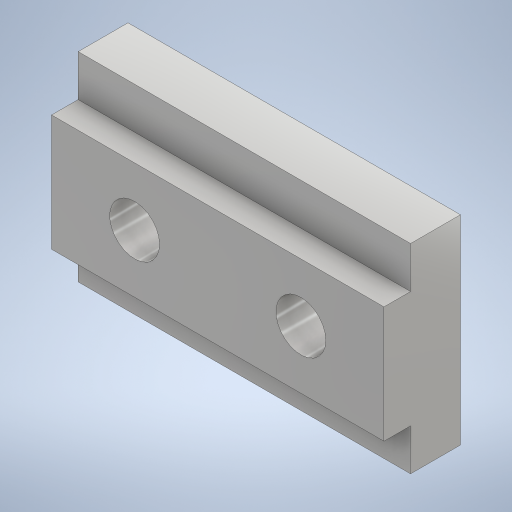
# Autodesk Inventor part: slider2b
Saved by Autodesk Inventor 2024.1 (Build 281209000, 209)
## iProperties
Created: 2017-08-05
Part Number: slider2b
Material: アルミニウム 6061-AHC
Document SubType Name: Modeling
Designer: SHUICHI
Density: 2.7 g/cm^3
Appearance: アルミニウム - ダーク
Mass: 2.37322 g
Surface Area: 8.16834 cm^2
Volume: 0.878969 cm^3
Author: SHUICHI
Autodesk Inventor part; units mm, degrees
ref_plane "YZ Plane" through (0, 0, 0) normal (1, 0, 0) x (0, 1, 0)
ref_plane "XZ Plane" through (0, 0, 0) normal (0, 1, 0) x (-1, 0, 0)
ref_plane "XY Plane" through (0, 0, 0) normal (0, 0, 1) x (1, 0, 0)
sketch "スケッチ1" plane through (0, 0, 0) normal (1, 0, 0) x (0, 1, 0)
  line L0 (0, 0) -> (1.6, 0)
  line L1 (1.6, 0) -> (1.6, 2.5)
  line L2 (1.6, 2.5) -> (4.6, 2.5)
  line L3 (4.6, 2.5) -> (4.6, -9.5)
  line L4 (4.6, -9.5) -> (1.6, -9.5)
  line L5 (1.6, -9.5) -> (1.6, -7)
  line L6 (1.6, -7) -> (0, -7)
  line L7 (0, -7) -> (0, 0)
  dimension "d0" = 4.6
  dimension "d1" = 7
  dimension "d2" = 12
  dimension "d3" = 2.5
  dimension "d4" = 3
  constraints: 16 end point, 6 perpendicular, 2 point on line, 1 horizontal
  measures "d0" distance between parallel lines of L7 L3
  measures "d1" distance of L6.end L0.start
  measures "d2" distance of L2.end L3.end
  measures "d3" distance of L0.end L1.end
  measures "d4" distance of L1.end L2.end
extrude "押し出し1" add sketch "スケッチ1" along normal blind 20
sketch "スケッチ2" plane through (0, 0, -7) normal (0, -1, 0) x (1, 0, 0)
  circle A0 centre (5, 3.5) radius 1.5
  circle A1 centre (15, 3.5) radius 1.5
  line L0 (0, 0) -> (0, 7) projected
  point P0 (0, 3.5)
  dimension "d7" = 3
  dimension "d8" = 3
  dimension "d9" = 5
  dimension "d10" = 10
  constraints: 2 centre point, 2 horizontal alignment, 1 midpoint
  measures "d7" diameter of A0
  measures "d8" diameter of A1
  measures "d9" distance from line of L0 A0.centre
  measures "d10" distance of A0.centre A1.centre
extrude "押し出し2" cut sketch "スケッチ2" against normal through all
